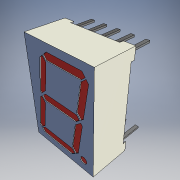
# Autodesk Inventor part: SA52-11EWA
Saved by Autodesk Inventor 2018 (Build 220112000, 112)
## iProperties
Created: 2020-04-20
Part Number: SA52-11EWA
Material: Všeobecné
Document SubType Name: Modeling
Designer: Jozko Mrkvicka
Density: 1 g/cm^3
Appearance: Výchozí
Author: Jozko Mrkvicka
Autodesk Inventor part; units mm, degrees
ref_plane "YZ Plane" through (0, 0, 0) normal (1, 0, 0) x (0, 1, 0)
ref_plane "XZ Plane" through (0, 0, 0) normal (0, 1, 0) x (-1, 0, 0)
ref_plane "XY Plane" through (0, 0, 0) normal (0, 0, 1) x (1, 0, 0)
sketch "Náčrt1" plane through (0, 0, 0) normal (0, 1, 0) x (-1, 0, 0)
  line L0 (0, 0) -> (17.78, 0)
  line L1 (17.78, 0) -> (17.78, -12.7)
  line L2 (17.78, -12.7) -> (0, -12.7)
  line L3 (0, -12.7) -> (0, 0)
  dimension "d0" = 17.78
  dimension "d1" = 12.7
  constraints: 8 end point, 2 parallel, 1 horizontal, 1 perpendicular
  measures "d0" distance of L1.end L2.end
  measures "d1" distance of L0.end L1.end
extrude "Vysunutí1" add sketch "Náčrt1" along normal blind 6.35
sketch "Náčrt2" plane through (0, 0, 0) normal (0, -1, 0) x (1, 0, 0)
  line L0 (0, 0) -> (0, -1.9143)
  line L1 (0, -1.9143) -> (-1.9143, 0)
  line L2 (0, 0) -> (-1.9143, 0)
  line L3 (-17.78, -12.7) -> (-17.78, -10.7857)
  line L4 (-17.78, -10.7857) -> (-15.8657, -12.7)
  line L5 (-17.78, -12.7) -> (-15.8657, -12.7)
  line L6 (0, -12.7) -> (-1.9143, -12.7)
  line L7 (-1.9143, -12.7) -> (0, -10.7857)
  line L8 (0, -12.7) -> (0, -10.7857)
  line L9 (-17.78, 0) -> (-15.8657, 0)
  line L10 (-15.8657, 0) -> (-17.78, -1.9143)
  line L11 (-17.78, 0) -> (-17.78, -1.9143)
  dimension "d4" = 45
  dimension "d5" = 45
  dimension "d6" = 45
  dimension "d7" = 45
  constraints: 24 end point, 1 horizontal, 1 vertical
  measures "d4" angle of L0 L1
  measures "d5" angle of L3 L4
  measures "d6" angle of L6 L7
  measures "d7" angle of L9 L10
extrude "Vysunutí2" add sketch "Náčrt2" along normal blind 0.635
sketch "Náčrt3" plane through (0, 0, 0) normal (0, -1, 0) x (1, 0, 0)
  line L0 (-16.3513, -0.9525) -> (-16.3513, -1.5875)
  line L1 (-16.3513, -1.5875) -> (-16.6687, -1.5875)
  line L2 (-16.6687, -1.5875) -> (-16.6688, -0.9525)
  line L3 (-16.6688, -0.9525) -> (-16.3513, -0.9525)
  line L4 (-16.3513, -3.4925) -> (-16.3513, -4.1275)
  line L5 (-16.3513, -4.1275) -> (-16.6687, -4.1275)
  line L6 (-16.6687, -4.1275) -> (-16.6688, -3.4925)
  line L7 (-16.6688, -3.4925) -> (-16.3513, -3.4925)
  line L8 (-16.3513, -6.0325) -> (-16.3513, -6.6675)
  line L9 (-16.3513, -6.6675) -> (-16.6687, -6.6675)
  line L10 (-16.6687, -6.6675) -> (-16.6688, -6.0325)
  line L11 (-16.6688, -6.0325) -> (-16.3513, -6.0325)
  line L12 (-16.3513, -8.5725) -> (-16.3513, -9.2075)
  line L13 (-16.3513, -9.2075) -> (-16.6687, -9.2075)
  line L14 (-16.6687, -9.2075) -> (-16.6688, -8.5725)
  line L15 (-16.6688, -8.5725) -> (-16.3513, -8.5725)
  line L16 (-16.3513, -11.1125) -> (-16.3513, -11.7475)
  line L17 (-16.3513, -11.7475) -> (-16.6687, -11.7475)
  line L18 (-16.6687, -11.7475) -> (-16.6688, -11.1125)
  line L19 (-16.6688, -11.1125) -> (-16.3513, -11.1125)
  line L20 (-1.1113, -0.9525) -> (-1.1113, -1.5875)
  line L21 (-1.1113, -1.5875) -> (-1.4288, -1.5875)
  line L22 (-1.4288, -1.5875) -> (-1.4288, -0.9525)
  line L23 (-1.4288, -0.9525) -> (-1.1113, -0.9525)
  line L24 (-1.1113, -3.4925) -> (-1.1113, -4.1275)
  line L25 (-1.1113, -4.1275) -> (-1.4288, -4.1275)
  line L26 (-1.4288, -4.1275) -> (-1.4288, -3.4925)
  line L27 (-1.4288, -3.4925) -> (-1.1113, -3.4925)
  line L28 (-1.1113, -6.0325) -> (-1.1113, -6.6675)
  line L29 (-1.1113, -6.6675) -> (-1.4288, -6.6675)
  line L30 (-1.4288, -6.6675) -> (-1.4288, -6.0325)
  line L31 (-1.4288, -6.0325) -> (-1.1113, -6.0325)
  line L32 (-1.1113, -8.5725) -> (-1.1113, -9.2075)
  line L33 (-1.1113, -9.2075) -> (-1.4288, -9.2075)
  line L34 (-1.4288, -9.2075) -> (-1.4288, -8.5725)
  line L35 (-1.4288, -8.5725) -> (-1.1113, -8.5725)
  line L36 (-1.1113, -11.1125) -> (-1.1112, -11.7475)
  line L37 (-1.1112, -11.7475) -> (-1.4287, -11.7475)
  line L38 (-1.4287, -11.7475) -> (-1.4288, -11.1125)
  line L39 (-1.4288, -11.1125) -> (-1.1113, -11.1125)
  point P0 (0, 0)
  point P1 (-16.51, -6.35)
  point P2 (-1.27, -6.35)
  point P3 (-16.51, -3.81)
  point P4 (-16.51, -8.89)
  point P5 (-1.27, -8.89)
  point P6 (-1.27, -3.81)
  point P7 (-16.51, -1.27)
  point P8 (-16.51, -3.81)
  point P9 (-16.51, -6.35)
  point P10 (-16.51, -8.89)
  point P11 (-16.51, -11.43)
  point P12 (-1.27, -1.27)
  point P13 (-1.27, -3.81)
  point P14 (-1.27, -6.35)
  point P15 (-1.27, -8.89)
  point P16 (-1.27, -11.43)
  constraints: 80 end point, 20 parallel, 10 perpendicular
extrude "Vysunutí3" add sketch "Náčrt3" along normal blind 5.08
sketch "Náčrt4" plane through (0, 0, 0) normal (0, -1, 0) x (1, 0, 0)
  line L0 (-1.1113, -9.2075) -> (-1.4288, -9.2075) projected
  line L1 (-1.4288, -9.2075) -> (-1.4288, -8.5725) projected
  line L2 (-1.4288, -8.5725) -> (-1.1113, -8.5725) projected
  line L3 (-1.1113, -8.5725) -> (-1.1113, -9.2075) projected
  line L4 (-1.1113, -4.1275) -> (-1.4288, -4.1275) projected
  line L5 (-1.4288, -4.1275) -> (-1.4288, -3.4925) projected
  line L6 (-1.4288, -3.4925) -> (-1.1113, -3.4925) projected
  line L7 (-1.1113, -3.4925) -> (-1.1113, -4.1275) projected
  line L8 (-16.3513, -11.7475) -> (-16.6687, -11.7475) projected
  line L9 (-16.6687, -11.7475) -> (-16.6688, -11.1125) projected
  line L10 (-16.6688, -11.1125) -> (-16.3513, -11.1125) projected
  line L11 (-16.3513, -11.1125) -> (-16.3513, -11.7475) projected
  line L12 (-16.3513, -6.6675) -> (-16.6687, -6.6675) projected
  line L13 (-16.6687, -6.6675) -> (-16.6688, -6.0325) projected
  line L14 (-16.6688, -6.0325) -> (-16.3513, -6.0325) projected
  line L15 (-16.3513, -6.0325) -> (-16.3513, -6.6675) projected
  line L16 (-16.3513, -1.5875) -> (-16.6687, -1.5875) projected
  line L17 (-16.6687, -1.5875) -> (-16.6688, -0.9525) projected
  line L18 (-16.6688, -0.9525) -> (-16.3513, -0.9525) projected
  line L19 (-16.3513, -0.9525) -> (-16.3513, -1.5875) projected
  line L20 (-16.3513, -4.1275) -> (-16.6687, -4.1275) projected
  line L21 (-16.6687, -4.1275) -> (-16.6688, -3.4925) projected
  line L22 (-16.6688, -3.4925) -> (-16.3513, -3.4925) projected
  line L23 (-16.3513, -3.4925) -> (-16.3513, -4.1275) projected
  line L24 (-16.3513, -9.2075) -> (-16.6687, -9.2075) projected
  line L25 (-16.6687, -9.2075) -> (-16.6688, -8.5725) projected
  line L26 (-16.6688, -8.5725) -> (-16.3513, -8.5725) projected
  line L27 (-16.3513, -8.5725) -> (-16.3513, -9.2075) projected
  line L28 (-1.1113, -1.5875) -> (-1.4288, -1.5875) projected
  line L29 (-1.4288, -1.5875) -> (-1.4288, -0.9525) projected
  line L30 (-1.4288, -0.9525) -> (-1.1113, -0.9525) projected
  line L31 (-1.1113, -0.9525) -> (-1.1113, -1.5875) projected
  line L32 (-1.1113, -6.6675) -> (-1.4288, -6.6675) projected
  line L33 (-1.4288, -6.6675) -> (-1.4288, -6.0325) projected
  line L34 (-1.4288, -6.0325) -> (-1.1113, -6.0325) projected
  line L35 (-1.1113, -6.0325) -> (-1.1113, -6.6675) projected
  line L36 (-1.1112, -11.7475) -> (-1.4287, -11.7475) projected
  line L37 (-1.4287, -11.7475) -> (-1.4288, -11.1125) projected
  line L38 (-1.4288, -11.1125) -> (-1.1113, -11.1125) projected
  line L39 (-1.1113, -11.1125) -> (-1.1112, -11.7475) projected
  line L40 (-1.9143, -12.7) -> (0, -10.7857) projected
  line L41 (0, -10.7857) -> (0, -1.9143) projected
  line L42 (0, -1.9143) -> (-1.9143, 0) projected
  line L43 (-1.9143, 0) -> (-15.8657, 0) projected
  line L44 (-17.78, -1.9143) -> (-17.78, -10.7857) projected
  line L45 (-17.78, -10.7857) -> (-15.8657, -12.7) projected
  line L46 (-15.8657, -12.7) -> (-1.9143, -12.7) projected
  line L47 (-3.81, -12.7) -> (-3.81, -12.3825)
  line L48 (-0.3175, -12.3825) -> (-17.6212, -12.3825)
  line L49 (0, -10.16) -> (-0.3175, -10.16)
  line L50 (-4.445, 0) -> (-4.445, -0.3175)
  line L51 (-17.78, -2.54) -> (-17.4625, -2.54)
  line L52 (-0.3175, -12.3825) -> (-0.3175, -1.5968)
  line L53 (-17.4625, -12.3825) -> (-17.4625, -1.5968)
  line L54 (-15.8657, -12.7) -> (-17.78, -10.7857) projected
  line L55 (-17.4625, -11.1032) -> (-16.1832, -12.3825)
  line L56 (-1.5968, -12.3825) -> (-0.3175, -11.1032)
  line L57 (-17.4625, -1.5968) -> (-16.1832, -0.3175)
  line L58 (-1.9143, 0) -> (0, -1.9143) projected
  line L59 (-17.4625, -1.5968) -> (-16.1832, -0.3175)
  line L60 (-17.78, -1.9143) -> (-15.8657, 0) projected
  line L61 (-1.5968, -0.3175) -> (-0.3175, -1.5968)
  line L62 (-1.5968, -0.3175) -> (-16.1832, -0.3175)
  line L63 (-17.4625, -0.3175) -> (-17.6212, -0.3175)
  point P0 (0, 0)
  constraints: 28 end point, 16 point on line, 3 horizontal, 3 parallel, 3 vertical, 2 collinear
extrude "Vysunutí4" cut sketch "Náčrt4" against normal blind 1.27 contours L48 L45 L53 L57 L62 L42 L52 L40
sketch "Náčrt5" plane through (0, 6.35, 0) normal (0, 1, 0) x (1, 0, 0)
  line L0 (-1.27, 8.255) -> (-1.27, 1.905)
  line L1 (-16.51, 4.445) -> (-16.51, 10.795)
  line L2 (-1.905, 8.9958) -> (-1.27, 8.255)
  line L3 (-1.905, 8.9958) -> (-2.54, 8.4667)
  line L4 (-1.27, 1.905) -> (-1.905, 1.3758)
  line L5 (-1.905, 1.3758) -> (-2.54, 2.1167)
  line L6 (-8.255, 3.0692) -> (-8.89, 2.54)
  line L7 (-8.89, 2.54) -> (-9.525, 3.2808)
  line L8 (-8.255, 9.4192) -> (-8.89, 10.16)
  line L9 (-8.89, 10.16) -> (-9.525, 9.6308)
  line L10 (-16.51, 10.795) -> (-15.875, 11.3242)
  line L11 (-15.24, 10.5833) -> (-15.875, 11.3242)
  line L12 (-2.8575, 8.5196) -> (-2.0611, 9.1832)
  line L13 (-2.8575, 2.1696) -> (-2.0637, 1.2435)
  line L14 (-15.24, 4.2333) -> (-15.875, 3.7042)
  line L15 (-15.875, 3.7042) -> (-16.51, 4.445)
  line L16 (-14.9225, 10.5304) -> (-15.7162, 11.4565)
  line L17 (-14.9151, 4.1792) -> (-15.7032, 3.5037)
  line L18 (-15.7162, 11.4565) -> (-15.24, 11.8533)
  line L19 (-15.7032, 3.5037) -> (-15.24, 2.9633)
  line L20 (-9.1768, 2.2942) -> (-9.525, 2.0108)
  line L21 (-8.6659, 2.2785) -> (-8.255, 1.7992)
  line L22 (-9.0982, 10.4098) -> (-9.525, 10.9008)
  line L23 (-8.5997, 10.4019) -> (-8.255, 10.6892)
  line L24 (-2.0637, 1.2435) -> (-2.54, 0.8467)
  line L25 (-2.0611, 9.1832) -> (-2.5195, 9.7333)
  line L26 (-2.54, 2.1167) -> (-2.54, 8.4667)
  line L27 (-2.8575, 2.1696) -> (-7.8267, 2.9978)
  line L28 (-9.525, 3.2808) -> (-9.525, 9.6308)
  line L29 (-7.8267, 2.9978) -> (-8.6659, 2.2785)
  line L30 (-15.24, 2.9633) -> (-9.525, 2.0108)
  line L31 (-8.255, 1.7992) -> (-2.54, 0.8467)
  line L32 (-10.16, 3.3867) -> (-9.1768, 2.2942)
  line L33 (-2.8575, 8.5196) -> (-7.62, 9.3133)
  line L34 (-8.255, 9.4192) -> (-8.255, 3.0692)
  line L35 (-2.5195, 9.7333) -> (-8.255, 10.6892)
  line L36 (-8.5997, 10.4019) -> (-7.62, 9.3133)
  line L37 (-9.9483, 9.7014) -> (-9.0982, 10.4098)
  line L38 (-9.9483, 9.7014) -> (-14.9225, 10.5304)
  line L39 (-9.525, 10.9008) -> (-15.24, 11.8533)
  line L40 (-10.16, 3.3867) -> (-14.9151, 4.1792)
  line L41 (-15.24, 4.2333) -> (-15.24, 10.5833)
  circle A0 centre (-15.875, 1.905) radius 0.635
  constraints: 84 end point, 10 parallel, 6 point on line, 3 perpendicular, 1 centre point
extrude "Vysunutí5" cut sketch "Náčrt5" against normal blind 0.127
